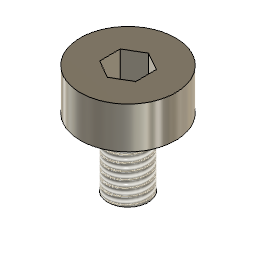
Rim Screw (Autodesk Fusion 360 design; units mm, degrees)
Autodesk Fusion 360 part; units mm, degrees
note: some values were not read from the file. Chosen so that the rebuilt part matches the saved one: how an offset face is resized. Set by a fixed rule: which face or edge a step refers to.
sketch "Sketch1" plane through (0, 0, 0) normal (0, 0, 1) x (1, 0, 0)
  circle A0 centre (0, 0) radius 4.6
  circle A1 centre (0, 0) radius 2
  line L0 (1.7394, -0.9872) -> (1.7246, 1.0128)
  line L1 (1.7246, 1.0128) -> (-0.0148, 1.9999)
  line L2 (-0.0148, 1.9999) -> (-1.7394, 0.9872)
  line L3 (-1.7394, 0.9872) -> (-1.7246, -1.0128)
  line L4 (-1.7246, -1.0128) -> (0.0148, -1.9999)
  line L5 (0.0148, -1.9999) -> (1.7394, -0.9872)
  dimension "d1" = 9.2
  dimension "d2" = 4
  constraint coincident A0.centre A1.centre
  constraint concentric A0 A1
  constraint coincident A1 L0.start
  measures "d1" diameter of A0
  measures "d2" diameter of A1
extrude "Extrude1" add sketch "Sketch1" against normal blind 6.5 contours A1 L0 | A1 L1 | L0 L1 L2 L3 L4 L5 | A1 L5 | A1 L2 | A1 L4 | A1 L3 makes body 1
extrude "Extrude2" add sketch "Sketch1" along normal blind 4 separate body contours A0 | A1 L0 | A1 L1 | A1 L5 | A1 L2 | A1 L4 | A1 L3 makes body 2
thread "Thread1" "ISO Metric profile 4.0 M4x0.7 M4x0.7 6g" major diameter 3.908 minor diameter 3.111 pitch 0.7 angle 60 resizes the face on face at (0.0849, 1.9982, -4.3333) on bodies 1
combine "Combine1" operation add target body 1 tool bodies 2
